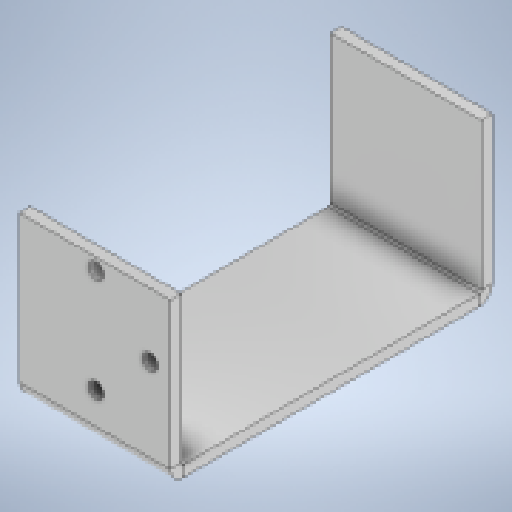
# Autodesk Inventor part: axis_25_bottom_frame
Saved by Autodesk Inventor 2025.2 (Build 292293000, 293)
## iProperties
Created: 2025-06-30
Part Number: axis_25_bottom_frame
Material: Aluminum 6061-AHC
Document SubType Name: Sheet Metal
Designer: LG
Density: 2.7 g/cm^3
Sheet Metal Rule: Default_mm
Appearance: Aluminum - Dark
Author: LG
Autodesk Inventor part; units mm, degrees
ref_plane "YZ Plane" through (0, 0, 0) normal (1, 0, 0) x (0, 1, 0)
ref_plane "XZ Plane" through (0, 0, 0) normal (0, 1, 0) x (-1, 0, 0)
ref_plane "XY Plane" through (0, 0, 0) normal (0, 0, 1) x (1, 0, 0)
sketch "Sketch1" plane through (0, 0, 0) normal (0, 1, 0) x (-1, 0, 0)
  line L0 (10.17, 20.25) -> (-9.97, 20.25)
  line L1 (-9.97, 20.25) -> (-9.97, -20.25)
  line L2 (-9.97, -20.25) -> (10.17, -20.25)
  line L3 (10.17, -20.25) -> (10.17, 20.25)
  point P0 (0, 0)
  dimension "d0" = 40.5
  dimension "d1" = 20.14
  dimension "d2" = 10.17
  dimension "d3" = 20.25
  measures "d0" distance of L2.end L0.start
  measures "d1" distance of L1.end L2.end
  measures "d2" distance from line of point (0, 0) L3
  measures "d3" distance from line of point (0, 0) L2
extrude "Plate1" add sketch "Sketch1" along normal blind 1.5
sketch "Sketch2" plane through (9.97, 0, 21.75) normal (0, 0, -1) x (-1, 0, 0)
  line L0 (20.14, 0) -> (0, 0)
  line L1 (0, 0) -> (0, 21.9)
  line L2 (0, 21.9) -> (20.14, 21.9)
  line L3 (20.14, 21.9) -> (20.14, 0)
  constraints: 8 end point
edge flange "Flange1" height 21.9 angle 90 thickness 1.5 bend radius 0.31 thickness toward (0, 0, -1) relief straight relief width 1.5 relief depth 0.75 corner gap 0.31 corner form 0 edges at (-0.1, 1.5, 20.25) (-0.1, 1.5, -20.25) wall of the first edge with corners at (-10.17, 0, 21.75) (9.97, 0, 21.75) (9.97, 21.9, 21.75) (-10.17, 21.9, 21.75)
bend "Bend1"
corner "Corner1"
sketch "Sketch3" plane through (-10.17, 21.9, 21.75) normal (0, 0, 1) x (1, 0, 0)
  circle A0 centre (10.16, -1.83) radius 0.7835 projected
  circle A1 centre (10.16, -15.83) radius 0.7835 projected
  circle A2 centre (17.46, -8.83) radius 0.7835 projected
  point P0 (10.17, -21.9)
hole "Hole1" at (-0.01, 20.07, 21.75) at (7.29, 13.07, 21.75) at (-0.01, 6.07, 21.75) direction (0, 0, -1) diameter 2.1 depth 1.5
sketch "Sketch4" plane through (9.97, 21.9, -21.75) normal (0, 0, -1) x (-1, 0, 0)
  circle A0 centre (2.5, -16.355) radius 0.7835 projected
  circle A1 centre (17.6, -16.355) radius 0.7835 projected
  circle A2 centre (17.6, -1.305) radius 0.7835 projected
  circle A3 centre (2.5, -1.305) radius 0.7835 projected
  point P0 (9.97, -21.9)
hole "Hole2" at (-7.63, 20.595, -21.75) at (-7.63, 5.545, -21.75) at (7.47, 5.545, -21.75) at (7.47, 20.595, -21.75) direction (0, 0, 1) diameter 2.1 depth 1.5
equation "\"d20\" = Thickness"
equation "\"d27\" = Thickness"
equation "\"d4\" = Thickness"
equation "\"d5\" = BendReliefWidth"
equation "\"d6\" = BendReliefDepth"
equation "\"d7\" = MinimumRemnant"
equation "\"d8\" = TransitionRadius"
equation "\"d11\" = BendRadius"
equation "\"d12\" = CornerReliefSize"
equation "\"d13\" = GapSize"
equation "\"d14\" = JacobiRadiusSize"
equation "\"BendReliefWidth\" = Thickness"
equation "\"BendReliefDepth\" = 0.5 * Thickness"
equation "\"CornerReliefSize\" = 4 * Thickness"
equation "\"MinimumRemnant\" = 2 * Thickness"
equation "\"TransitionRadius\" = BendRadius"
equation "\"JacobiRadiusSize\" = BendRadius"
equation "\"GapSize\" = Thickness"
equation "\"Thickness\" = 1.5"
equation "\"BendRadius\" = 0.31"
body "Solid1"
